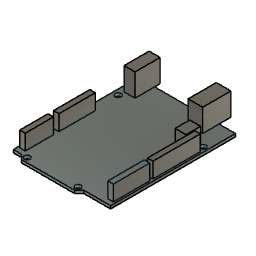
arduinoUNO v1 (Autodesk Fusion 360 design; units mm, degrees)
Autodesk Fusion 360 part; units mm, degrees
sketch "Sketch1" plane through (0, 0, 0) normal (0, 0, 1) x (1, 0, 0)
  line L0 (-52.4, 1.3) -> (1, 1.3)
  line L1 (1, 1.3) -> (1, -67.3)
  line L2 (1, -67.3) -> (-52.4, -67.3)
  line L3 (-52.4, -67.3) -> (-52.4, 1.3)
  dimension "d1" = 68.6
  dimension "d2" = 53.4
  constraint horizontal L0
  constraint vertical L1
  constraint horizontal L2
  constraint vertical L3
  measures "d1" distance of L0.start L2.end
  measures "d2" distance of L1.end L2.end
extrude "Extrude1" add sketch "Sketch1" along normal blind 1.6
sketch "Sketch3" plane through (0, 0, 1.6) normal (0, 0, 1) x (-1, 0, 0)
  line L0 (52.4, 67.3) -> (-1, 67.3)
  line L1 (-1, 67.3) -> (-1, -1.3)
  line L2 (-1, -1.3) -> (52.4, -1.3)
  line L3 (52.4, -1.3) -> (52.4, 67.3)
  line L4 (3, 64.76) -> (0, 64.76)
  line L5 (0, 64.76) -> (0, 44.76)
  line L6 (0, 44.76) -> (3, 44.76)
  line L7 (3, 44.76) -> (3, 64.76)
  dimension "d5" = 20
  dimension "d6" = 2.54
  dimension "d7" = 3
  dimension "d34" = 1
  constraint horizontal L4
  constraint vertical L5
  constraint horizontal L6
  constraint vertical L7
  measures "d5" distance of L4.start L6.end
  measures "d6" distance of L0 L4
  measures "d7" distance of L5.end L6.end
  measures "d34" distance of L1 L5
extrude "Extrude2" add sketch "Sketch3" along normal blind 8.5 contours L4 L5 L6 L7
sketch "Sketch4" plane through (0, 0, 1.6) normal (0, 0, 1) x (-1, 0, 0)
  line L0 (3, 44.76) -> (0, 44.76)
  line L1 (0, 44.76) -> (0, 64.76)
  line L2 (0, 64.76) -> (3, 64.76)
  line L3 (3, 64.76) -> (3, 44.76)
  line L4 (52.4, 67.3) -> (-1, 67.3)
  line L5 (-1, 67.3) -> (-1, -1.3)
  line L6 (-1, -1.3) -> (52.4, -1.3)
  line L7 (52.4, -1.3) -> (52.4, 67.3)
  line L8 (51.4, 49.26) -> (48.4, 49.26)
  line L9 (48.4, 49.26) -> (48.4, 64.76)
  line L10 (48.4, 64.76) -> (51.4, 64.76)
  line L11 (51.4, 64.76) -> (51.4, 49.26)
  dimension "d10" = 15.5
  dimension "d11" = 2.54
  dimension "d12" = 3
  dimension "d36" = 1
  constraint horizontal L8
  constraint vertical L9
  constraint horizontal L10
  constraint vertical L11
  measures "d10" distance of L8.end L9.end
  measures "d11" distance of L4 L10
  measures "d12" distance of L8.start L8.end
  measures "d36" distance of L7 L11
extrude "Extrude3" add sketch "Sketch4" along normal blind 8.5 contours L8 L9 L10 L11
sketch "Sketch5" plane through (0, 0, 1.6) normal (0, 0, 1) x (-1, 0, 0)
  line L0 (51.4, 64.76) -> (51.4, 49.26)
  line L1 (51.4, 49.26) -> (48.4, 49.26)
  line L2 (48.4, 49.26) -> (48.4, 64.76)
  line L3 (48.4, 64.76) -> (51.4, 64.76)
  line L4 (3, 44.76) -> (0, 44.76)
  line L5 (0, 44.76) -> (0, 64.76)
  line L6 (0, 64.76) -> (3, 64.76)
  line L7 (3, 64.76) -> (3, 44.76)
  line L8 (52.4, 67.3) -> (-1, 67.3)
  line L9 (-1, 67.3) -> (-1, -1.3)
  line L10 (-1, -1.3) -> (52.4, -1.3)
  line L11 (52.4, -1.3) -> (52.4, 67.3)
  line L12 (51.4, 26.26) -> (48.4, 26.26)
  line L13 (48.4, 26.26) -> (48.4, 46.26)
  line L14 (48.4, 46.26) -> (51.4, 46.26)
  line L15 (51.4, 46.26) -> (51.4, 26.26)
  dimension "d15" = 20
  dimension "d16" = 3
  dimension "d17" = 3
  dimension "d35" = 1
  constraint horizontal L12
  constraint vertical L13
  constraint horizontal L14
  constraint vertical L15
  measures "d15" distance of L12.start L14.end
  measures "d16" distance of L12.start L12.end
  measures "d17" distance of L1 L14
  measures "d35" distance of L11 L15
extrude "Extrude4" add sketch "Sketch5" along normal blind 8.5 contours L12 L13 L14 L15
sketch "Sketch6" plane through (0, 0, 1.6) normal (0, 0, 1) x (-1, 0, 0)
  line L0 (51.4, 46.26) -> (51.4, 26.26)
  line L1 (51.4, 26.26) -> (48.4, 26.26)
  line L2 (48.4, 26.26) -> (48.4, 46.26)
  line L3 (48.4, 46.26) -> (51.4, 46.26)
  line L4 (51.4, 64.76) -> (51.4, 49.26)
  line L5 (51.4, 49.26) -> (48.4, 49.26)
  line L6 (48.4, 49.26) -> (48.4, 64.76)
  line L7 (48.4, 64.76) -> (51.4, 64.76)
  line L8 (3, 44.76) -> (0, 44.76)
  line L9 (0, 44.76) -> (0, 64.76)
  line L10 (0, 64.76) -> (3, 64.76)
  line L11 (3, 64.76) -> (3, 44.76)
  line L12 (52.4, 67.3) -> (-1, 67.3)
  line L13 (-1, 67.3) -> (-1, -1.3)
  line L14 (-1, -1.3) -> (52.4, -1.3)
  line L15 (52.4, -1.3) -> (52.4, 67.3)
  line L16 (9.5, 13.3) -> (3.5, 13.3)
  line L17 (3.5, 13.3) -> (3.5, 21.3)
  line L18 (3.5, 21.3) -> (9.5, 21.3)
  line L19 (9.5, 21.3) -> (9.5, 13.3)
  dimension "d20" = 8
  dimension "d21" = 6
  dimension "d22" = 46
  dimension "d23" = 0.5
  constraint horizontal L16
  constraint vertical L17
  constraint horizontal L18
  constraint vertical L19
  measures "d20" distance of L16.start L18.end
  measures "d21" distance of L17.end L18.end
  measures "d22" distance of L12 L18
  measures "d23" distance of L11 L17
extrude "Extrude5" add sketch "Sketch6" along normal blind 8.5 contours L16 L17 L18 L19
sketch "Sketch7" plane through (0, 0, 1.6) normal (0, 0, 1) x (-1, 0, 0)
  line L0 (9.5, 21.3) -> (9.5, 13.3)
  line L1 (9.5, 13.3) -> (3.5, 13.3)
  line L2 (3.5, 13.3) -> (3.5, 21.3)
  line L3 (3.5, 21.3) -> (9.5, 21.3)
  line L4 (51.4, 46.26) -> (51.4, 26.26)
  line L5 (51.4, 26.26) -> (48.4, 26.26)
  line L6 (48.4, 26.26) -> (48.4, 46.26)
  line L7 (48.4, 46.26) -> (51.4, 46.26)
  line L8 (51.4, 64.76) -> (51.4, 49.26)
  line L9 (51.4, 49.26) -> (48.4, 49.26)
  line L10 (48.4, 49.26) -> (48.4, 64.76)
  line L11 (48.4, 64.76) -> (51.4, 64.76)
  line L12 (3, 44.76) -> (0, 44.76)
  line L13 (0, 44.76) -> (0, 64.76)
  line L14 (0, 64.76) -> (3, 64.76)
  line L15 (3, 64.76) -> (3, 44.76)
  line L16 (52.4, 67.3) -> (-1, 67.3)
  line L17 (-1, 67.3) -> (-1, -1.3)
  line L18 (-1, -1.3) -> (52.4, -1.3)
  line L19 (52.4, -1.3) -> (52.4, 67.3)
  circle A0 centre (1.5, 13.94) radius 1.6
  dimension "d26" = 3.2
  dimension "d27" = 15.24
  dimension "d28" = 2.5
  measures "d26" diameter of A0
  measures "d27" distance of L18 A0.centre
  measures "d28" distance of L17 A0.centre
sketch "Sketch8" plane through (0, 0, 10.1) normal (0, 0, 1) x (-1, 0, 0)
  line L0 (3, 44.76) -> (3, 64.76)
  line L1 (3, 64.76) -> (0, 64.76)
  line L2 (0, 64.76) -> (0, 44.76)
  line L3 (0, 44.76) -> (3, 44.76)
sketch "Sketch9" plane through (0, 0, 1.6) normal (0, 0, 1) x (1, 0, 0)
  line L0 (0, -43) -> (-3, -43)
  line L1 (-3, -43) -> (-3, -17)
  line L2 (-3, -17) -> (0, -17)
  line L3 (0, -17) -> (0, -43)
  line L4 (1, -67.3) -> (1, 1.3)
  dimension "d29" = 26
  dimension "d30" = 3
  dimension "d31" = 1
  constraint horizontal L0
  constraint vertical L1
  constraint horizontal L2
  constraint vertical L3
  measures "d29" distance of L0.start L2.end
  measures "d30" distance of L1.end L2.end
  measures "d31" distance of L3 L4
extrude "Extrude6" add sketch "Sketch9" along normal blind 8.5
extrude "Extrude7" cut sketch "Sketch7" against normal blind 50 contours A0
sketch "Sketch10" plane through (0, 0, 1.6) normal (0, 0, 1) x (-1, 0, 0)
  circle A0 centre (1.5, 13.94) radius 1.6
  line L0 (0, 17) -> (0, 43)
  line L1 (0, 43) -> (3, 43)
  line L2 (3, 43) -> (3, 17)
  line L3 (3, 17) -> (0, 17)
  line L4 (9.5, 21.3) -> (9.5, 13.3)
  line L5 (9.5, 13.3) -> (3.5, 13.3)
  line L6 (3.5, 13.3) -> (3.5, 21.3)
  line L7 (3.5, 21.3) -> (9.5, 21.3)
  line L8 (51.4, 46.26) -> (51.4, 26.26)
  line L9 (51.4, 26.26) -> (48.4, 26.26)
  line L10 (48.4, 26.26) -> (48.4, 46.26)
  line L11 (48.4, 46.26) -> (51.4, 46.26)
  line L12 (51.4, 64.76) -> (51.4, 49.26)
  line L13 (51.4, 49.26) -> (48.4, 49.26)
  line L14 (48.4, 49.26) -> (48.4, 64.76)
  line L15 (48.4, 64.76) -> (51.4, 64.76)
  line L16 (3, 44.76) -> (0, 44.76)
  line L17 (0, 44.76) -> (0, 64.76)
  line L18 (0, 64.76) -> (3, 64.76)
  line L19 (3, 64.76) -> (3, 44.76)
  line L20 (52.4, 67.3) -> (-1, 67.3)
  line L21 (-1, 67.3) -> (-1, -1.3)
  line L22 (-1, -1.3) -> (52.4, -1.3)
  line L23 (52.4, -1.3) -> (52.4, 67.3)
  line L24 (49.4, -4.3) -> (43.4, -4.3)
  line L25 (43.4, -4.3) -> (43.4, 9.47)
  line L26 (43.4, 9.47) -> (49.4, 9.47)
  line L27 (49.4, 9.47) -> (49.4, -4.3)
  dimension "d39" = 13.77
  dimension "d40" = 3
  dimension "d41" = 6
  dimension "d44" = 3
  constraint horizontal L24
  constraint vertical L25
  constraint horizontal L26
  constraint vertical L27
  measures "d39" distance of L24.start L26.end
  measures "d40" distance of L22 L24
  measures "d41" distance of L24.start L24.end
  measures "d44" distance of L23 L27
extrude "Extrude8" add sketch "Sketch10" along normal blind 12.5 contours L22 L24 L25 L27 | L22 L25 L26 L27
sketch "Sketch11" plane through (0, 0, 1.6) normal (0, 0, 1) x (-1, 0, 0)
  line L0 (49.4, 9.47) -> (49.4, -1.3)
  line L1 (49.4, -1.3) -> (52.4, -1.3)
  line L2 (52.4, -1.3) -> (52.4, 67.3)
  line L3 (52.4, 67.3) -> (-1, 67.3)
  line L4 (-1, 67.3) -> (-1, -1.3)
  line L5 (-1, -1.3) -> (43.4, -1.3)
  line L6 (43.4, -1.3) -> (43.4, 9.47)
  line L7 (43.4, 9.47) -> (49.4, 9.47)
  circle A0 centre (1.5, 13.94) radius 1.6
  line L8 (0, 17) -> (0, 43)
  line L9 (0, 43) -> (3, 43)
  line L10 (3, 43) -> (3, 17)
  line L11 (3, 17) -> (0, 17)
  line L12 (9.5, 21.3) -> (9.5, 13.3)
  line L13 (9.5, 13.3) -> (3.5, 13.3)
  line L14 (3.5, 13.3) -> (3.5, 21.3)
  line L15 (3.5, 21.3) -> (9.5, 21.3)
  line L16 (51.4, 46.26) -> (51.4, 26.26)
  line L17 (51.4, 26.26) -> (48.4, 26.26)
  line L18 (48.4, 26.26) -> (48.4, 46.26)
  line L19 (48.4, 46.26) -> (51.4, 46.26)
  line L20 (51.4, 64.76) -> (51.4, 49.26)
  line L21 (51.4, 49.26) -> (48.4, 49.26)
  line L22 (48.4, 49.26) -> (48.4, 64.76)
  line L23 (48.4, 64.76) -> (51.4, 64.76)
  line L24 (3, 44.76) -> (0, 44.76)
  line L25 (0, 44.76) -> (0, 64.76)
  line L26 (0, 64.76) -> (3, 64.76)
  line L27 (3, 64.76) -> (3, 44.76)
  circle A1 centre (49.5158, 12.67) radius 1.6
  dimension "d45" = 3.2
  dimension "d46" = 13.97
  measures "d45" diameter of A1
  measures "d46" distance of L1 A1.centre
extrude "Extrude9" cut sketch "Sketch11" against normal blind 1.6 contours A1
sketch "Sketch13" plane through (0, 0, 1.6) normal (0, 0, 1) x (-1, 0, 0)
  circle A0 centre (49.5158, 12.67) radius 1.6
  line L0 (49.4, 9.47) -> (49.4, -1.3)
  line L1 (49.4, -1.3) -> (52.4, -1.3)
  line L2 (52.4, -1.3) -> (52.4, 67.3)
  line L3 (52.4, 67.3) -> (-1, 67.3)
  line L4 (-1, 67.3) -> (-1, -1.3)
  line L5 (-1, -1.3) -> (43.4, -1.3)
  line L6 (43.4, -1.3) -> (43.4, 9.47)
  line L7 (43.4, 9.47) -> (49.4, 9.47)
  circle A1 centre (1.5, 13.94) radius 1.6
  line L8 (0, 17) -> (0, 43)
  line L9 (0, 43) -> (3, 43)
  line L10 (3, 43) -> (3, 17)
  line L11 (3, 17) -> (0, 17)
  line L12 (9.5, 21.3) -> (9.5, 13.3)
  line L13 (9.5, 13.3) -> (3.5, 13.3)
  line L14 (3.5, 13.3) -> (3.5, 21.3)
  line L15 (3.5, 21.3) -> (9.5, 21.3)
  line L16 (51.4, 46.26) -> (51.4, 26.26)
  line L17 (51.4, 26.26) -> (48.4, 26.26)
  line L18 (48.4, 26.26) -> (48.4, 46.26)
  line L19 (48.4, 46.26) -> (51.4, 46.26)
  line L20 (51.4, 64.76) -> (51.4, 49.26)
  line L21 (51.4, 49.26) -> (48.4, 49.26)
  line L22 (48.4, 49.26) -> (48.4, 64.76)
  line L23 (48.4, 64.76) -> (51.4, 64.76)
  line L24 (3, 44.76) -> (0, 44.76)
  line L25 (0, 44.76) -> (0, 64.76)
  line L26 (0, 64.76) -> (3, 64.76)
  line L27 (3, 64.76) -> (3, 44.76)
  line L28 (-1, 69.84) -> (52, 69.84)
  line L29 (13.64, 67.3) -> (16.1805, 69.84)
  line L30 (45.429, 69.84) -> (47.97, 67.3)
  dimension "d49" = 2.54
  dimension "d50" = 14.64
  dimension "d51" = 4.43
  constraint horizontal L28
  constraint coincident L3 L29.start
  constraint coincident L28 L29.end
  constraint coincident L28 L30.start
  constraint coincident L3 L30.end
  measures "d49" distance of L3 L28
  measures "d50" distance of L3.end L29.start
  measures "d51" distance of L2.end L30.end
extrude "Extrude10" add sketch "Sketch13" against normal blind 1.6 contours L3 L28 L29 L30
sketch "Sketch14" plane through (0, 0, 1.6) normal (0, 0, 1) x (-1, 0, 0)
  circle A0 centre (49.5158, 12.67) radius 1.6
  line L0 (49.4, 9.47) -> (49.4, -1.3)
  line L1 (49.4, -1.3) -> (52.4, -1.3)
  line L2 (52.4, -1.3) -> (52.4, 67.3)
  line L3 (52.4, 67.3) -> (47.97, 67.3)
  line L4 (47.97, 67.3) -> (45.429, 69.84)
  line L5 (45.429, 69.84) -> (16.1805, 69.84)
  line L6 (16.1805, 69.84) -> (13.64, 67.3)
  line L7 (13.64, 67.3) -> (-1, 67.3)
  line L8 (-1, 67.3) -> (-1, -1.3)
  line L9 (-1, -1.3) -> (43.4, -1.3)
  line L10 (43.4, -1.3) -> (43.4, 9.47)
  line L11 (43.4, 9.47) -> (49.4, 9.47)
  circle A1 centre (1.5, 13.94) radius 1.6
  line L12 (0, 17) -> (0, 43)
  line L13 (0, 43) -> (3, 43)
  line L14 (3, 43) -> (3, 17)
  line L15 (3, 17) -> (0, 17)
  line L16 (9.5, 21.3) -> (9.5, 13.3)
  line L17 (9.5, 13.3) -> (3.5, 13.3)
  line L18 (3.5, 13.3) -> (3.5, 21.3)
  line L19 (3.5, 21.3) -> (9.5, 21.3)
  line L20 (51.4, 46.26) -> (51.4, 26.26)
  line L21 (51.4, 26.26) -> (48.4, 26.26)
  line L22 (48.4, 26.26) -> (48.4, 46.26)
  line L23 (48.4, 46.26) -> (51.4, 46.26)
  line L24 (51.4, 64.76) -> (51.4, 49.26)
  line L25 (51.4, 49.26) -> (48.4, 49.26)
  line L26 (48.4, 49.26) -> (48.4, 64.76)
  line L27 (48.4, 64.76) -> (51.4, 64.76)
  line L28 (3, 44.76) -> (0, 44.76)
  line L29 (0, 44.76) -> (0, 64.76)
  line L30 (0, 64.76) -> (3, 64.76)
  line L31 (3, 64.76) -> (3, 44.76)
  circle A2 centre (16.84, 67.3) radius 1.6
  dimension "d54" = 3.2
  dimension "d55" = 17.84
  dimension "d56" = 2.54
  measures "d54" diameter of A2
  measures "d55" horizontal distance of L7.end A2.centre
  measures "d56" distance of L5 A2.centre
sketch "Sketch15" plane through (0, 0, 1.6) normal (0, 0, 1) x (1, 0, 0)
  circle A0 centre (-44.77, -67.3) radius 1.6
  line L0 (-45.429, -69.84) -> (-16.1805, -69.84)
  point P0 (-52.4, -67.3)
  dimension "d57" = 3.2
  dimension "d58" = 7.63
  dimension "d59" = 2.54
  measures "d57" diameter of A0
  measures "d58" horizontal distance of A0.centre P0
  measures "d59" distance of A0.centre L0
extrude "Extrude11" cut sketch "Sketch14" against normal blind 1.6 contours A2
extrude "Extrude12" cut sketch "Sketch15" against normal blind 1.6
sketch "Sketch16" plane through (0, 0, 1.6) normal (0, 0, 1) x (-1, 0, 0)
  circle A0 centre (44.77, 67.3) radius 1.6
  circle A1 centre (16.84, 67.3) radius 1.6
  circle A2 centre (49.5158, 12.67) radius 1.6
  line L0 (49.4, 9.47) -> (49.4, -1.3)
  line L1 (49.4, -1.3) -> (52.4, -1.3)
  line L2 (52.4, -1.3) -> (52.4, 67.3)
  line L3 (52.4, 67.3) -> (47.97, 67.3)
  line L4 (47.97, 67.3) -> (45.429, 69.84)
  line L5 (45.429, 69.84) -> (16.1805, 69.84)
  line L6 (16.1805, 69.84) -> (13.64, 67.3)
  line L7 (13.64, 67.3) -> (-1, 67.3)
  line L8 (-1, 67.3) -> (-1, -1.3)
  line L9 (-1, -1.3) -> (43.4, -1.3)
  line L10 (43.4, -1.3) -> (43.4, 9.47)
  line L11 (43.4, 9.47) -> (49.4, 9.47)
  circle A3 centre (1.5, 13.94) radius 1.6
  line L12 (0, 17) -> (0, 43)
  line L13 (0, 43) -> (3, 43)
  line L14 (3, 43) -> (3, 17)
  line L15 (3, 17) -> (0, 17)
  line L16 (9.5, 21.3) -> (9.5, 13.3)
  line L17 (9.5, 13.3) -> (3.5, 13.3)
  line L18 (3.5, 13.3) -> (3.5, 21.3)
  line L19 (3.5, 21.3) -> (9.5, 21.3)
  line L20 (51.4, 46.26) -> (51.4, 26.26)
  line L21 (51.4, 26.26) -> (48.4, 26.26)
  line L22 (48.4, 26.26) -> (48.4, 46.26)
  line L23 (48.4, 46.26) -> (51.4, 46.26)
  line L24 (51.4, 64.76) -> (51.4, 49.26)
  line L25 (51.4, 49.26) -> (48.4, 49.26)
  line L26 (48.4, 49.26) -> (48.4, 64.76)
  line L27 (48.4, 64.76) -> (51.4, 64.76)
  line L28 (3, 44.76) -> (0, 44.76)
  line L29 (0, 44.76) -> (0, 64.76)
  line L30 (0, 64.76) -> (3, 64.76)
  line L31 (3, 64.76) -> (3, 44.76)
  line L32 (8, 7.7) -> (16, 7.7)
  line L33 (16, 7.7) -> (16, -7.8)
  line L34 (16, -7.8) -> (8, -7.8)
  line L35 (8, -7.8) -> (8, 7.7)
  dimension "d64" = 15.5
  dimension "d65" = 9
  constraint horizontal L32
  constraint vertical L33
  constraint horizontal L34
  constraint vertical L35
  measures "d64" distance of L32.start L34.end
  measures "d65" distance of L9 L32
extrude "Extrude13" add sketch "Sketch16" along normal blind 12.5 contours L9 L33 L34 L35 | L9 L32 L33 L35
sketch "Sketch17" plane through (0, 0, 1.6) normal (0, 0, 1) x (-1, 0, 0)
  line L0 (16, 7.7) -> (16, -1.3)
  line L1 (16, -1.3) -> (43.4, -1.3)
  line L2 (43.4, -1.3) -> (43.4, 9.47)
  line L3 (43.4, 9.47) -> (49.4, 9.47)
  line L4 (49.4, 9.47) -> (49.4, -1.3)
  line L5 (49.4, -1.3) -> (52.4, -1.3)
  line L6 (52.4, -1.3) -> (52.4, 67.3)
  line L7 (52.4, 67.3) -> (47.97, 67.3)
  line L8 (47.97, 67.3) -> (45.429, 69.84)
  line L9 (45.429, 69.84) -> (16.1805, 69.84)
  line L10 (16.1805, 69.84) -> (13.64, 67.3)
  line L11 (13.64, 67.3) -> (-1, 67.3)
  line L12 (-1, 67.3) -> (-1, -1.3)
  line L13 (-1, -1.3) -> (8, -1.3)
  line L14 (8, -1.3) -> (8, 7.7)
  line L15 (8, 7.7) -> (16, 7.7)
  circle A0 centre (44.77, 67.3) radius 1.6
  circle A1 centre (16.84, 67.3) radius 1.6
  circle A2 centre (49.5158, 12.67) radius 1.6
  circle A3 centre (1.5, 13.94) radius 1.6
  line L16 (0, 17) -> (0, 43)
  line L17 (0, 43) -> (3, 43)
  line L18 (3, 43) -> (3, 17)
  line L19 (3, 17) -> (0, 17)
  line L20 (9.5, 21.3) -> (9.5, 13.3)
  line L21 (9.5, 13.3) -> (3.5, 13.3)
  line L22 (3.5, 13.3) -> (3.5, 21.3)
  line L23 (3.5, 21.3) -> (9.5, 21.3)
  line L24 (51.4, 46.26) -> (51.4, 26.26)
  line L25 (51.4, 26.26) -> (48.4, 26.26)
  line L26 (48.4, 26.26) -> (48.4, 46.26)
  line L27 (48.4, 46.26) -> (51.4, 46.26)
  line L28 (51.4, 64.76) -> (51.4, 49.26)
  line L29 (51.4, 49.26) -> (48.4, 49.26)
  line L30 (48.4, 49.26) -> (48.4, 64.76)
  line L31 (48.4, 64.76) -> (51.4, 64.76)
  line L32 (3, 44.76) -> (0, 44.76)
  line L33 (0, 44.76) -> (0, 64.76)
  line L34 (0, 64.76) -> (3, 64.76)
  line L35 (3, 64.76) -> (3, 44.76)
